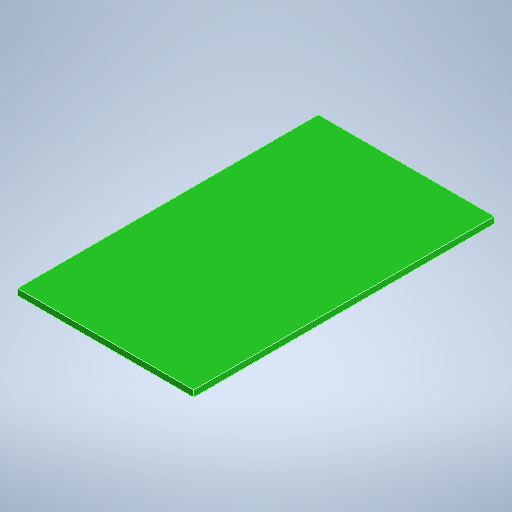
# Autodesk Inventor part: plytka
Saved by Autodesk Inventor 2025 (Build 290162000, 162)
## iProperties
Created: 2026-04-03
Part Number: plytka
Material: Miedź
Document SubType Name: Modeling
Designer: zzapa
Density: 8.94 g/cm^3
Appearance: Ogólny
Author: zzapa
Autodesk Inventor part; units mm, degrees
ref_plane "YZ Plane" through (0, 0, 0) normal (1, 0, 0) x (0, 1, 0)
ref_plane "XZ Plane" through (0, 0, 0) normal (0, 1, 0) x (-1, 0, 0)
ref_plane "XY Plane" through (0, 0, 0) normal (0, 0, 1) x (1, 0, 0)
sketch "Szkic1" plane through (0, 0, 0) normal (0, 1, 0) x (-1, 0, 0)
  line L0 (41, -70) -> (0, -70)
  line L1 (0, -70) -> (0, 0)
  line L2 (0, 0) -> (41, 0)
  line L3 (41, 0) -> (41, -70)
  dimension "d0" = 70
  dimension "d1" = 41
  constraints: 8 end point, 2 parallel, 1 horizontal, 1 perpendicular
  measures "d0" distance of L2.end L0.start
  measures "d1" distance of L0.start L0.end
extrude "Wyciągnięcie proste1" add sketch "Szkic1" along normal blind 1.5
